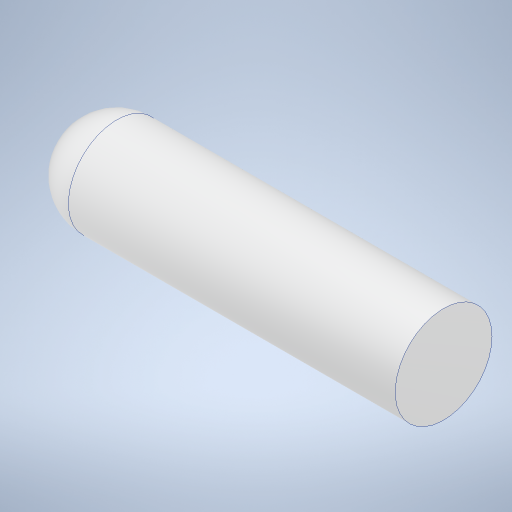
# Autodesk Inventor part: VierDurchmesser_Bolz
Saved by Autodesk Inventor 2024 (Build 280153000, 153)
## iProperties
Created: 2024-03-07
Part Number: VierDurchmesser_Bolz
Material: Aluminium 6061
Document SubType Name: Modeling
Designer: ffogue
Density: 2.7 g/cm^3
Appearance: Aluminium - flach
Author: ffogue
Autodesk Inventor part; units mm, degrees
ref_plane "YZ Plane" through (0, 0, 0) normal (1, 0, 0) x (0, 1, 0)
ref_plane "XZ Plane" through (0, 0, 0) normal (0, 1, 0) x (-1, 0, 0)
ref_plane "XY Plane" through (0, 0, 0) normal (0, 0, 1) x (1, 0, 0)
sketch "Skizze1" plane through (0, 0, 0) normal (0, 0, 1) x (1, 0, 0)
  line L0 (0, 0) -> (15.5, 0)
  line L1 (15.5, 0) -> (15.5, 2)
  line L2 (15.5, 2) -> (2, 2)
  arc A0 (2, 2) -> (0, 0) centre (2, 0) ccw
  dimension "d0" = 15.5
  dimension "d1" = 4
  constraints: 6 end point, 2 point on circle, 1 centre point, 1 coincident, 1 horizontal, 1 horizontal alignment, 1 perpendicular, 1 tangent, 1 vertical
  measures "d0" distance of L0.start L0.end
  measures "d1" diameter of L2 L0
revolve "Umdrehung1" add sketch "Skizze1" angle 360 about axis through (0, 0, 0) along (1, 0, 0)
